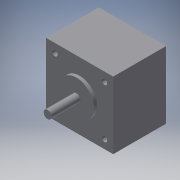
# Autodesk Inventor part: stepper
Saved by Autodesk Inventor 2019.4 (Build 234330000, 330)
## iProperties
Created: 2021-03-26
Part Number: stepper
Material: Generic
Document SubType Name: Modeling
Designer: Ian
Density: 1 g/cm^3
Appearance: Default
Author: Ian
Autodesk Inventor part; units mm, degrees
ref_plane "YZ Plane" through (0, 0, 0) normal (1, 0, 0) x (0, 1, 0)
ref_plane "XZ Plane" through (0, 0, 0) normal (0, 1, 0) x (-1, 0, 0)
ref_plane "XY Plane" through (0, 0, 0) normal (0, 0, 1) x (1, 0, 0)
sketch "Sketch1" plane through (0, 0, 0) normal (0, 0, 1) x (1, 0, 0)
  circle A0 centre (0, 0) radius 2.5
  line L0 (-15.5, 15.5) -> (15.5, 15.5) construction
  line L1 (15.5, 15.5) -> (15.5, -15.5) construction
  line L2 (15.5, -15.5) -> (-15.5, -15.5) construction
  line L3 (-15.5, -15.5) -> (-15.5, 15.5) construction
  line L4 (-15.5, 15.5) -> (15.5, -15.5) construction
  circle A1 centre (-15.5, 15.5) radius 1.75
  circle A2 centre (15.5, 15.5) radius 1.75
  circle A3 centre (15.5, -15.5) radius 1.75
  circle A4 centre (-15.5, -15.5) radius 1.75
  line L5 (-21, 21) -> (21, 21)
  line L6 (21, 21) -> (21, -21)
  line L7 (21, -21) -> (-21, -21)
  line L8 (-21, -21) -> (-21, 21)
  line L9 (-21, -21) -> (21, 21) construction
  dimension "d0" = 5
  dimension "d1" = 31
  dimension "d2" = 3.5
  dimension "d3" = 42
  constraints: 20 end point, 7 coincident, 5 centre point, 4 parallel, 4 perpendicular, 3 equal radius, 2 horizontal, 2 midpoint
  measures "d0" diameter of A0
  measures "d1" distance of L0.start L0.end
  measures "d2" diameter of A1
  measures "d3" distance of L5.start L5.end
extrude "Extrusion1" add sketch "Sketch1" against normal blind 33 contours A0 | L5 L6 L7 L8
extrude "Extrusion2" add sketch "Sketch1" along normal blind 20 contours A0
sketch "Sketch2" plane through (0, 0, 0) normal (0, 0, 1) x (1, 0, 0)
  circle A0 centre (0, 0) radius 11
  dimension "d8" = 22
  constraints: 1 centre point, 1 coincident
  measures "d8" diameter of A0
extrude "Extrusion3" add sketch "Sketch2" along normal blind 2
sketch "Sketch3" plane through (0, 0, 20) normal (0, 0, 1) x (1, 0, 0)
  circle A0 centre (0, 0) radius 2.5 projected
  line L0 (-1.5, 2) -> (1.5, 2)
  circle A1 centre (0, 0) radius 2.5 projected
  arc A2 (1.5, 2) -> (-1.5, 2) centre (0, 0) ccw
  dimension "d11" = 4.5
  constraints: 3 point on circle, 2 end point, 1 centre point, 1 concentric, 1 horizontal, 2 other
extrude "Extrusion4" cut sketch "Sketch3" against normal up to surface (18 mm away) contours L0 A0 picked at (-0.3466, 2.0912)
sketch "Sketch4" plane through (0, 0, 0) normal (0, 0, 1) x (1, 0, 0)
  circle A0 centre (-15.5, 15.5) radius 1.75 projected
  circle A1 centre (-15.5, 15.5) radius 3
  circle A2 centre (15.5, 15.5) radius 1.75 projected
  circle A3 centre (15.5, 15.5) radius 3
  point P0 (0, 0)
  dimension "d14" = 6
  dimension "d15" = 6
  constraints: 2 centre point, 2 coincident
  measures "d14" diameter of A1
  measures "d15" diameter of A3
body "Solid1"
